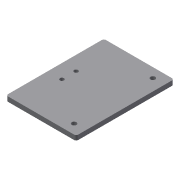
# Autodesk Inventor part: Neje_Sidewall_0
Saved by Autodesk Inventor 2019.4 (Build 234330000, 330)
## iProperties
Created: 2021-04-08
Part Number: Neje_Sidewall_0
Material: Generic
Document SubType Name: Modeling
Designer: diederichbenedict
Density: 1 g/cm^3
Appearance: Black
Author: diederichbenedict
Autodesk Inventor part; units mm, degrees
ref_plane "YZ Plane" through (0, 0, 0) normal (1, 0, 0) x (0, 1, 0)
ref_plane "XZ Plane" through (0, 0, 0) normal (0, 1, 0) x (-1, 0, 0)
ref_plane "XY Plane" through (0, 0, 0) normal (0, 0, 1) x (1, 0, 0)
sketch "Sketch1" plane through (0, 0, 0) normal (0, 1, 0) x (-1, 0, 0)
  line L0 (2, 0) -> (67.64, 0)
  line L1 (69.64, -2) -> (69.64, -95.15)
  line L2 (67.64, -97.15) -> (2, -97.15)
  line L3 (0, -95.15) -> (0, -2)
  circle A0 centre (11.5, -9.5) radius 2.355
  circle A1 centre (11.5, -87.65) radius 2.355
  arc A2 (69.64, -2) -> (67.64, 0) centre (67.64, -2) ccw
  arc A3 (67.64, -97.15) -> (69.64, -95.15) centre (67.64, -95.15) ccw
  arc A4 (2, 0) -> (0, -2) centre (2, -2) ccw
  arc A5 (0, -95.15) -> (2, -97.15) centre (2, -95.15) ccw
  circle A6 centre (55.64, -41.5) radius 2
  circle A7 centre (55.64, -55.55) radius 2
  point P0 (0, 0)
  point P1 (69.64, -97.15)
  point P2 (69.64, 0)
  point P3 (0, -97.15)
  dimension "d0" = 69.64
  dimension "d1" = 97.15
  dimension "d2" = 4.71
  dimension "d3" = 4.71
  dimension "d4" = 9.5
  dimension "d5" = 9.5
  dimension "d6" = 11.5
  dimension "d7" = 11.5
  dimension "d8" = 2
  dimension "d9" = 4
  dimension "d10" = 4
  dimension "d11" = 14
  dimension "d12" = 14
  dimension "d13" = 41.5
  dimension "d14" = 41.6
  constraints: 8 centre point, 8 end point, 8 point on circle, 8 point on line, 8 tangent, 3 equal radius, 2 parallel, 1 horizontal, 1 perpendicular
  measures "d0" distance of point (69.64, -97.15) point (0, -97.15)
  measures "d1" distance of point (69.64, 0) point (69.64, -97.15)
  measures "d2" diameter of A0
  measures "d3" diameter of A1
  measures "d4" distance from line of A0.centre L0
  measures "d5" distance from line of L2 A1.centre
  measures "d6" distance from line of A1.centre L3
  measures "d7" distance from line of A0.centre L3
  measures "d8" radius of A2
  measures "d9" diameter of A6
  measures "d10" diameter of A7
  measures "d11" distance from line of A6.centre L1
  measures "d12" distance from line of A7.centre L1
  measures "d13" distance from line of A6.centre L0
  measures "d14" distance from line of A7.centre L2
extrude "Extrusion1" add sketch "Sketch1" along normal blind 4.66
body "Solid1"
